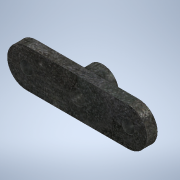
# Autodesk Inventor part: lab_3_1
Saved by Autodesk Inventor 2020 (Build 240168000, 168)
## iProperties
Created: 2020-03-17
Part Number: lab_3_1
Material: Сталь
Document SubType Name: Modeling
Designer: User
Density: 7.85 g/cm^3
Appearance: Листовая
Author: User
Autodesk Inventor part; units mm, degrees
ref_plane "YZ Plane" through (0, 0, 0) normal (1, 0, 0) x (0, 1, 0)
ref_plane "XZ Plane" through (0, 0, 0) normal (0, 1, 0) x (-1, 0, 0)
ref_plane "XY Plane" through (0, 0, 0) normal (0, 0, 1) x (1, 0, 0)
sketch "Эскиз1" plane through (0, 0, 0) normal (0, 0, 1) x (1, 0, 0)
  arc A0 (40, -15) -> (40, 15) centre (40, 0) ccw
  line L0 (40, -15) -> (-40, -15)
  arc A1 (-40, 15) -> (-40, -15) centre (-40, 0) ccw
  line L1 (-40, 15) -> (40, 15)
  circle A2 centre (-40, 0) radius 5
  circle A3 centre (40, 0) radius 5
  circle A4 centre (0, 0) radius 12.5
  circle A5 centre (0, 0) radius 6
  point P0 (0, 0)
  dimension "d2" = 80
  dimension "d6" = 10
  dimension "d7" = 10
  dimension "d9" = 25
  dimension "d10" = 12
  constraints: 6 centre point, 4 end point, 4 point on circle, 3 tangent, 2 coincident, 1 horizontal
  measures "d2" distance of L0.start L0.end
  measures "d6" diameter of A2
  measures "d7" diameter of A3
  measures "d9" diameter of A4
  measures "d10" diameter of A5
extrude "Выдавливание1" add sketch "Эскиз1" along normal blind 8 contours L0 A1 L1 A0 | A2 | A3 | A4 | A5
extrude "Выдавливание2" cut sketch "Эскиз1" along normal blind 8 contours A2
extrude "Выдавливание3" cut sketch "Эскиз1" along normal blind 8 contours A3
extrude "Выдавливание4" add sketch "Эскиз1" against normal blind 12 contours A4
extrude "Выдавливание5" cut sketch "Эскиз1" along normal blind 12 contours A5
